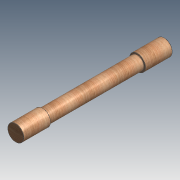
# Autodesk Inventor part: mallet_new
Saved by Autodesk Inventor 2015 (Build 190159000, 159)
## iProperties
Created: 2014-08-31
Part Number: mallet_new
Material: Wood (Birch)
Document SubType Name: Modeling
Designer: shohei
Density: 0.55 g/cm^3
Appearance: Birch - Natural Polished
Author: shohei
Autodesk Inventor part; units mm, degrees
ref_plane "YZ Plane" through (0, 0, 0) normal (1, 0, 0) x (0, 1, 0)
ref_plane "XZ Plane" through (0, 0, 0) normal (0, 1, 0) x (-1, 0, 0)
ref_plane "XY Plane" through (0, 0, 0) normal (0, 0, 1) x (1, 0, 0)
sketch "Sketch1" plane through (0, 0, 0) normal (0, 1, 0) x (-1, 0, 0)
  circle A0 centre (0, 0) radius 60
  dimension "d0" = 120
  constraints: 1 centre point, 1 coincident
  measures "d0" diameter of A0
extrude "Extrusion1" add sketch "Sketch1" along normal blind 200
sketch "Sketch2" plane through (0, 200, 0) normal (0, 1, 0) x (1, 0, 0)
  circle A0 centre (0, 0) radius 50
  dimension "d3" = 100
  constraints: 1 centre point, 1 coincident
  measures "d3" diameter of A0
extrude "Extrusion2" add sketch "Sketch2" along normal blind 700
sketch "Sketch3" plane through (0, 900, 0) normal (0, 1, 0) x (1, 0, 0)
  circle A0 centre (0, 0) radius 60
  dimension "d6" = 120
  constraints: 1 centre point, 1 coincident
  measures "d6" diameter of A0
extrude "Extrusion3" add sketch "Sketch3" along normal blind 200
fillet "Fillet1" radius 2 1 edges at (60, 200, 0)
fillet "Fillet2" radius 2 1 edges at (-50, 200, 0)
fillet "Fillet3" radius 2 2 edges at (-60, 900, 0) (-50, 900, 0)
fillet "Fillet4" radius 2 1 edges at (-60, 1100, 0)
fillet "Fillet5" radius 2 1 edges at (60, 0, 0)
equation "\"d1\" = 2 * Grip"
equation "\"d3\" = Grip"
equation "\"d4\" = 7 * Grip"
equation "\"d7\" = 2 * Grip"
equation "\"Grip\" = 100"
body "Solid1"
